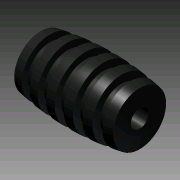
# Autodesk Inventor part: Roller Ridges 1764
Saved by Autodesk Inventor 2011 (Build 150239000, 239)
## iProperties
Created: 2007-11-28
Part Number: Roller Ridges 1764
Document SubType Name: Modeling
Designer: lwoods
Density: 1.4 g/cm^3
Material: PVC-Piping
Mass: 16.1581 g
Surface Area: 36.0602 cm^2
Volume: 11.5415 cm^3
Author: lwoods
Autodesk Inventor part; units mm, degrees
ref_plane "YZ Plane" through (0, 0, 0) normal (1, 0, 0) x (0, 1, 0)
ref_plane "XZ Plane" through (0, 0, 0) normal (0, 1, 0) x (-1, 0, 0)
ref_plane "XY Plane" through (0, 0, 0) normal (0, 0, 1) x (1, 0, 0)
sketch "Sketch1" plane through (0, 0, 0) normal (0, 0, 1) x (1, 0, 0)
  line L0 (-20.3007, 0.313) -> (-20.3007, -6.037)
  line L1 (-20.3007, -6.037) -> (15.2593, -6.037)
  line L2 (15.2593, -6.037) -> (15.2593, 0.313)
  line L3 (-25.6296, -9.212) -> (23.1111, -9.212)
  line L4 (-0.9332, 1.9649) -> (-0.9332, -0.3846)
  line L5 (-0.9332, -0.3846) -> (-4.1082, -0.3846)
  line L6 (-4.1082, -0.3846) -> (-4.1082, 1.9649)
  line L7 (-13.8466, 1.306) -> (-13.8466, -1.4757)
  line L8 (-13.8466, -1.4757) -> (-17.0216, -1.4757)
  line L9 (-17.0216, -1.4757) -> (-17.0216, 0.8738)
  line L10 (11.9801, 0.8738) -> (11.9801, -1.4757)
  line L11 (11.9801, -1.4757) -> (8.8051, -1.4757)
  line L12 (8.8051, -1.4757) -> (8.8051, 1.306)
  line L13 (-7.3925, 1.8541) -> (-7.3925, -0.7101)
  line L14 (-7.3925, -0.7101) -> (-10.5675, -0.7101)
  line L15 (-10.5675, -0.7101) -> (-10.5675, 1.6394)
  line L16 (5.526, 1.6394) -> (5.526, -0.7101)
  line L17 (5.526, -0.7101) -> (2.351, -0.7101)
  line L18 (2.351, -0.7101) -> (2.351, 1.8541)
  arc A0 (-17.0216, 0.8738) -> (-20.3007, 0.313) centre (-2.5207, -93.7799) ccw
  arc A1 (-10.5675, 1.6394) -> (-13.8466, 1.306) centre (-2.5207, -93.7799) ccw
  arc A2 (-4.1082, 1.9649) -> (-7.3925, 1.8541) centre (-2.5207, -93.7799) ccw
  arc A3 (2.351, 1.8541) -> (-0.9332, 1.9649) centre (-2.5207, -93.7799) ccw
  arc A4 (15.2593, 0.313) -> (11.9801, 0.8738) centre (-2.5207, -93.7799) ccw
  arc A5 (8.8051, 1.306) -> (5.526, 1.6394) centre (-2.5207, -93.7799) ccw
  dimension "d0" = 35.56
  dimension "d1" = 6.35
  dimension "d2" = 6.35
  dimension "d4" = 3.175
  dimension "d7" = 3.175
  dimension "d10" = 3.2791
  dimension "d11" = 3.175
  dimension "d13" = 3.2791
  dimension "d16" = 3.2791
  dimension "d18" = 3.2791
  dimension "d19" = 16.1925
  dimension "d20" = 3.175
  dimension "d21" = 3.175
  dimension "d22" = 3.175
  dimension "d23" = 2.3495
  dimension "d24" = 2.3495
  dimension "d25" = 2.3495
  dimension "d26" = 2.3495
  dimension "d27" = 2.3495
  dimension "d28" = 7.7363
  dimension "d29" = 8.502
  dimension "d30" = 8.8275
  constraints: 38 end point, 12 point on circle, 6 centre point, 6 parallel, 2 perpendicular, 1 vertical
  measures "d0" distance of L0.end L1.end
  measures "d1" distance of L0.start L0.end
  measures "d2" distance of L1.end L2.end
  measures "d4" distance between parallel lines of L1 L3
  measures "d7" distance between parallel lines of L4 L6
  measures "d10" distance between parallel lines of L0 L9
  measures "d11" distance between parallel lines of L13 L15
  measures "d13" distance between parallel lines of L15 L7
  measures "d16" distance between parallel lines of L12 L16
  measures "d18" distance between parallel lines of L2 L10
  measures "d19" distance between parallel lines of L6 L0
  measures "d20" distance of L16.end L17.end
  measures "d21" distance of L10.end L11.end
  measures "d22" distance of L7.end L8.end
  measures "d23" distance of L4.start L4.end
  measures "d24" distance of L16.start L16.end
  measures "d25" distance of L10.start L10.end
  measures "d26" distance of L14.end L15.end
  measures "d27" distance of L8.end L9.end
  measures "d28" distance between parallel lines of L3 L8
  measures "d29" distance between parallel lines of L3 L14
  measures "d30" distance between parallel lines of L3 L5
revolve "Revolution1" add sketch "Sketch1" angle 360 about axis through (-25.6296, -9.212, 0) along (1, 0, 0)
body "Solid1"
